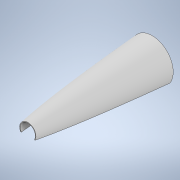
# Autodesk Inventor part: nose-toppart1
Saved by Autodesk Inventor 2020.3 (Build 243373000, 373)
## iProperties
Created: 2021-03-10
Part Number: nose-toppart1
Material: Generic
Document SubType Name: Modeling
Designer: 0x6f736f646f
Density: 1 g/cm^3
Appearance: Default
Mass: 19.8997 g
Surface Area: 280.653 cm^2
Volume: 19.8997 cm^3
Author: 0x6f736f646f
Autodesk Inventor part; units mm, degrees
ref_plane "YZ Plane" through (0, 0, 0) normal (1, 0, 0) x (0, 1, 0)
ref_plane "XZ Plane" through (0, 0, 0) normal (0, 1, 0) x (-1, 0, 0)
ref_plane "XY Plane" through (0, 0, 0) normal (0, 0, 1) x (1, 0, 0)
sketch "Sketch3" plane through (0, 0, 0) normal (1, 0, 0) x (0, 1, 0)
  line L0 (0, 0) -> (26.8, 0)
  line L1 (26.8, 0) -> (26.8, -5)
  line L2 (26.8, -5) -> (28.6, -5)
  line L3 (28.6, -5) -> (28.6, 0)
  line L4 (0, 0) -> (-26.8, 0)
  line L5 (-26.8, 0) -> (-26.8, -5)
  line L6 (-26.8, -5) -> (-28.6, -5)
  line L7 (-28.6, -5) -> (-28.6, 0)
  line L8 (0, 0) -> (0, 200)
  line L9 (0, 0) -> (0, 198.2)
  line L10 (0, 0) -> (0, 170)
  spline S0 degree 2 poles (28.6, 0) (0, 400) (-28.6, 0) knots 0 0 0 1 1 1
  spline S1 degree 2 poles (26.8, 0) (0, 396.4) (-26.8, 0) knots 0 0 0 1 1 1
  line L11 (0, 2) -> (28.4566, 2)
  line L12 (0, 170) -> (11.0767, 170)
  line L13 (0, 172) -> (10.7011, 172)
  line L14 (0, 0) -> (-5, 0)
  line L15 (-5, 0) -> (-5, 170)
  line L16 (-5, 170) -> (0, 170)
  line L17 (0, 170) -> (0, 0)
  line L18 (-5, 0) -> (-15, 0)
  line L19 (-15, 0) -> (-5, 170)
  line L20 (0, -46.4) -> (0, 243.4)
  line L21 (0, 2) -> (-28.4566, 2)
  line L22 (0, -104.36) -> (0, 301.36) projected
  point P0 (-1.8, 200)
  point P1 (9.0895, 172)
  point P2 (0, 172)
  point P3 (9.43, 170)
  point P4 (24.8735, 2)
  point P5 (0, 2)
  point P6 (0, 170)
  point P7 (9.7439, 172)
  point P8 (10.109, 170)
  point P9 (26.6644, 2)
  point P10 (-14.8824, 2)
  point P11 (10.109, 170)
  point P12 (26.6644, 2)
  point P13 (-14.8824, 2)
  dimension "d37" = 26.8
  dimension "d38" = 5
  dimension "d39" = 1.8
  dimension "d40" = 26.8
  dimension "d41" = 5
  dimension "d42" = 1.8
  dimension "d43" = 200
  dimension "d44" = 198.2
  dimension "d45" = 170
  dimension "d46" = 2
  dimension "d47" = 2
  dimension "d48" = 5
  dimension "d49" = 10
  dimension "d50" = 86.633
  constraints: 44 end point, 7 perpendicular, 6 point on line, 5 horizontal, 4 parallel, 1 collinear, 1 vertical, 10 other
  measures "d37" distance of L0.start L0.end
  measures "d38" distance of L0.end L1.end
  measures "d39" distance of L1.end L2.end
  measures "d40" distance of L0.start L4.end
  measures "d41" distance of L4.end L5.end
  measures "d42" distance of L5.end L6.end
  measures "d43" distance of L0.start L8.end
  measures "d44" distance of L0.start L9.end
  measures "d45" distance of L0.start L10.end
  measures "d46" distance between parallel lines of L0 L11
  measures "d47" distance between parallel lines of L12 L13
  measures "d48" distance of L15.end L16.end
  measures "d49" distance of L14.end L18.end
  measures "d50" angle of L18 L19
revolve "Revolution4" add sketch "Sketch3" angle 360 mid plane about axis through (0, 0, -10) along (0, 0, 1) contours S1 L12 S0 L11
extrude "Extrusion4" cut sketch "Sketch3" along normal mid plane 60 contours L16 L19 L21 S1 L8 | L21 S0 L8 S1
body "Solid3"
